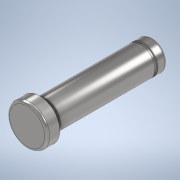
# Autodesk Inventor part: 6-鞘轴
Saved by Autodesk Inventor 2022 (Build 260153000, 153)
## iProperties
Created: 2023-01-08
Part Number: 6-鞘轴
Material: 不锈钢
Document SubType Name: Modeling
Designer: Lzy18
Density: 8 g/cm^3
Appearance: 半抛光
Author: Lzy18
Autodesk Inventor part; units mm, degrees
ref_plane "YZ Plane" through (0, 0, 0) normal (1, 0, 0) x (0, 1, 0)
ref_plane "XZ Plane" through (0, 0, 0) normal (0, 1, 0) x (-1, 0, 0)
ref_plane "XY Plane" through (0, 0, 0) normal (0, 0, 1) x (1, 0, 0)
sketch "草图1" plane through (0, 0, 0) normal (0, 1, 0) x (-1, 0, 0)
  line L0 (0, 0) -> (-8, 0)
  line L1 (-8, 0) -> (-8, -5)
  line L2 (-8, -5) -> (0, -5)
  line L3 (0, -5) -> (0, 0)
  line L4 (0, -5) -> (-5, -5)
  line L5 (-5, -5) -> (-5, -7.5)
  line L6 (-5, -7.5) -> (0, -7.5)
  line L7 (0, -7.5) -> (0, -5)
  line L8 (0, -7.5) -> (-5.75, -7.5)
  line L9 (-5.75, -7.5) -> (-5.75, -45)
  line L10 (-5.75, -45) -> (0, -45)
  line L11 (0, -45) -> (0, -7.5)
  line L12 (0, -45) -> (-5.25, -45)
  line L13 (-5.25, -45) -> (-5.25, -46.1)
  line L14 (-5.25, -46.1) -> (0, -46.1)
  line L15 (0, -46.1) -> (0, -45)
  line L16 (0, -46.1) -> (-5.75, -46.1)
  line L17 (-5.75, -46.1) -> (-5.75, -50)
  line L18 (-5.75, -50) -> (0, -50)
  line L19 (0, -50) -> (0, -46.1)
  dimension "d0" = 8
  dimension "d1" = 5
  dimension "d2" = 5
  dimension "d3" = 2.5
  dimension "d4" = 5.75
  dimension "d5" = 37.5
  dimension "d6" = 5.25
  dimension "d7" = 1.1
  dimension "d8" = 5.75
  dimension "d9" = 3.9
  constraints: 40 end point, 10 parallel, 5 horizontal, 5 perpendicular
  measures "d0" distance of L2.end L1.end
  measures "d1" distance of L1.end L0.end
  measures "d2" distance of L6.end L5.end
  measures "d3" distance of L5.end L4.end
  measures "d4" distance of L10.end L9.end
  measures "d5" distance of L9.end L8.end
  measures "d6" distance of L14.end L13.end
  measures "d7" distance of L13.end L12.end
  measures "d8" distance of L18.end L17.end
  measures "d9" distance of L17.end L16.end
revolve "旋转1" add sketch "草图1" angle 360 about axis through (0, 0, -45) along (0, 0, 1)
fillet "圆角1" radius 1 2 edges at (-8, 0, 0) (-5.75, 0, -50)
